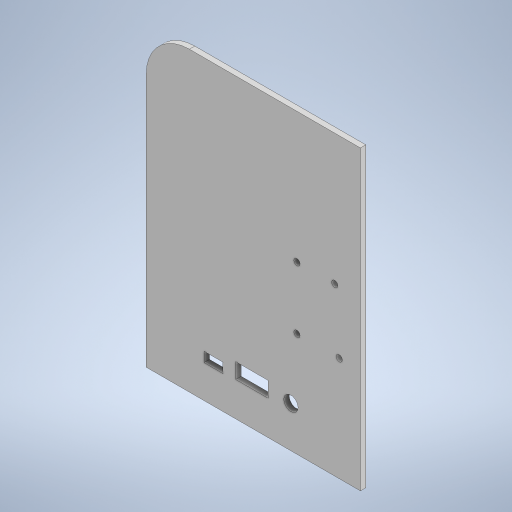
# Autodesk Inventor part: acrylicSidePanel
Saved by Autodesk Inventor 2023 (Build 270158000, 158)
## iProperties
Created: 2022-07-14
Part Number: acrylicSidePanel
Material: Generic
Document SubType Name: Modeling
Designer: Zain Ali
Density: 1 g/cm^3
Appearance: Default
Author: Zain Ali
Autodesk Inventor part; units mm, degrees
ref_plane "YZ Plane" through (0, 0, 0) normal (1, 0, 0) x (0, 1, 0)
ref_plane "XZ Plane" through (0, 0, 0) normal (0, 1, 0) x (-1, 0, 0)
ref_plane "XY Plane" through (0, 0, 0) normal (0, 0, 1) x (1, 0, 0)
sketch "Sketch1" plane through (0, 0, 0) normal (0, 0, 1) x (1, 0, 0)
  line L0 (0, 0) -> (-119, 0)
  line L1 (-119, 0) -> (-119, 165)
  line L2 (-119, 165) -> (0, 165)
  line L3 (0, 165) -> (0, 0)
  arc A0 (-95, 165) -> (-119, 141) centre (-95, 141) ccw
  dimension "d0" = 119
  dimension "d1" = 24
  dimension "d2" = 165
  constraints: 8 end point, 2 parallel, 2 point on circle, 2 point on line, 2 tangent, 1 centre point, 1 horizontal, 1 perpendicular
  measures "d0" distance of L0.start L0.end
  measures "d1" radius of A0
  measures "d2" distance of L2.end L0.start
extrude "Extrusion1" add sketch "Sketch1" along normal blind 3 contours L0 L1 A0 L2 L3
sketch "Sketch2" plane through (0, 0, 3) normal (0, 0, 1) x (1, 0, 0)
  circle A0 centre (-35.25, 92.45) radius 1.75
  circle A1 centre (-14.25, 92.45) radius 1.75
  circle A2 centre (-11.75, 57.95) radius 1.75
  circle A3 centre (-35.25, 57.95) radius 1.75
  circle A4 centre (-38.5965, 22.8) radius 3
  circle A5 centre (-38.5965, 22.8) radius 4
  line L0 (-69.2578, 27.53) -> (-51.2578, 27.53)
  line L1 (-51.2578, 27.53) -> (-51.2578, 18.98)
  line L2 (-51.2578, 18.98) -> (-69.2578, 18.98)
  line L3 (-69.2578, 18.98) -> (-69.2578, 27.53)
  line L4 (-67.7578, 25.23) -> (-67.7578, 22.7561)
  line L5 (-52.7578, 22.7561) -> (-52.7578, 25.23)
  line L6 (-53.5578, 26.03) -> (-66.9578, 26.03)
  line L7 (-59.8078, 20.48) -> (-55.4728, 20.48)
  line L8 (-77.8522, 21.65) -> (-77.8522, 20.9314)
  line L9 (-78.9836, 19.8) -> (-81.5993, 19.8)
  line L10 (-85.3522, 20.9314) -> (-85.3522, 21.65)
  line L11 (-84.7522, 22.25) -> (-78.4522, 22.25)
  line L12 (-86.8522, 23.75) -> (-76.3522, 23.75)
  line L13 (-76.3522, 23.75) -> (-76.3522, 18.3)
  line L14 (-76.3522, 18.3) -> (-86.8522, 18.3)
  line L15 (-86.8522, 18.3) -> (-86.8522, 23.75)
  line L16 (0, 0) -> (0, 165) projected
  line L17 (0, 165) -> (-95, 165) projected
  arc A6 (-95, 165) -> (-119, 141) centre (-95, 141) ccw projected
  line L18 (-119, 141) -> (-119, 0) projected
  line L19 (-119, 0) -> (0, 0) projected
  point P0 (-52.7578, 23.9931)
  dimension "d51" = 1
  dimension "d52" = 15
  dimension "d53" = 1.5
  dimension "d54" = 1.5
  dimension "d55" = 1.5
  dimension "d56" = 1.5
  dimension "d57" = 1.5
  dimension "d58" = 1.5
  dimension "d59" = 1.5
  dimension "d60" = 1.5
  dimension "d63" = 3.5
  dimension "d64" = 8
  dimension "d72" = 138.97
  dimension "d73" = 144.52
  dimension "d74" = 145.2
  dimension "d75" = 141.25
  dimension "d76" = 52.7578
  dimension "d77" = 76.3522
  dimension "d78" = 86.8522
  dimension "d82" = 67.7578
  dimension "d96" = 107.05
  dimension "d97" = 11.75
  dimension "d98" = 72.55
  dimension "d99" = 14.25
  dimension "d102" = 72.55
  dimension "d103" = 35.25
  dimension "d104" = 107.05
  dimension "d105" = 35.25
  dimension "d106" = 38.5965
  dimension "d107" = 139.77
  dimension "d108" = 141.0069
  dimension "d109" = 53.5578
  dimension "d110" = 55.4728
  dimension "d111" = 59.8078
  dimension "d112" = 66.9578
  dimension "d113" = 139.77
  dimension "d114" = 142.2439
  dimension "d115" = 143.35
  dimension "d116" = 144.0686
  dimension "d117" = 78.4522
  dimension "d118" = 78.9836
  dimension "d119" = 81.5993
  dimension "d120" = 84.7522
  dimension "d121" = 143.35
  dimension "d122" = 144.0686
  constraints: 32 end point, 8 parallel, 6 centre point, 3 equal radius, 2 horizontal, 2 perpendicular, 1 coincident, 1 midpoint, 1 tangent
  measures "d51" radial gap between concentric circles of A4 A5
  measures "d52" distance from line of point (-52.758, 23.993) L4
  measures "d53" horizontal distance of L5.end L0.end
  measures "d54" horizontal distance of L4.start L3.end
  measures "d55" distance from line of L0 L6.start
  measures "d56" distance from line of L2 L7.end
  measures "d57" distance between parallel lines of L13 L8
  measures "d58" distance between parallel lines of L12 L11
  measures "d59" distance between parallel lines of L9 L14
  measures "d60" distance between parallel lines of L15 L10
  measures "d63" diameter of A2
  measures "d64" diameter of A5
  measures "d72" distance between parallel lines of L17 L6
  measures "d73" distance between parallel lines of L17 L7
  measures "d74" distance between parallel lines of L17 L9
  measures "d75" distance between parallel lines of L17 L12
  measures "d76" distance between parallel lines of L16 L5
  measures "d77" distance between parallel lines of L16 L13
  measures "d78" distance between parallel lines of L16 L15
  measures "d82" distance between parallel lines of L4 L16
  measures "d96" distance from line of A2.centre L17
  measures "d97" distance from line of A2.centre L16
  measures "d98" distance from line of A1.centre L17
  measures "d99" distance from line of A1.centre L16
  measures "d102" distance from line of A0.centre L17
  measures "d103" distance from line of A0.centre L16
  measures "d104" distance from line of A3.centre L17
  measures "d105" distance from line of A3.centre L16
  measures "d106" distance from line of A4.centre L16
  measures "d107" distance from line of L5.end L17
  measures "d108" distance from line of point (-52.758, 23.993) L17
  measures "d109" distance from line of L6.start L16
  measures "d110" distance from line of L7.end L16
  measures "d111" distance from line of L7.start L16
  measures "d112" distance from line of L6.end L16
  measures "d113" distance from line of L4.start L17
  measures "d114" distance from line of L4.end L17
  measures "d115" distance from line of L8.start L17
  measures "d116" distance from line of L8.end L17
  measures "d117" distance from line of L11.end L16
  measures "d118" distance from line of L9.start L16
  measures "d119" distance from line of L9.end L16
  measures "d120" distance from line of L11.start L16
  measures "d121" distance from line of L10.end L17
  measures "d122" distance from line of L10.start L17
extrude "Extrusion2" cut sketch "Sketch2" against normal through all contours A0 | A1 | A2 | A3 | A4 | A5 | L0 L1 L2 L3 | L12 L13 L14 L15
body "Solid1"
